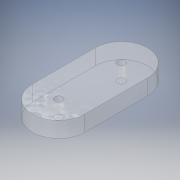
# Autodesk Inventor part: case_usb_cap
Saved by Autodesk Inventor 2019 (Build 230136000, 136)
## iProperties
Created: 2019-02-02
Part Number: case_usb_cap
Material: Acrylic, Clear
Document SubType Name: Modeling
Designer: suchanek
Density: 1.19 g/cm^3
Appearance: Transparent - Clear
Author: suchanek
Autodesk Inventor part; units mm, degrees
ref_plane "YZ Plane" through (0, 0, 0) normal (1, 0, 0) x (0, 1, 0)
ref_plane "XZ Plane" through (0, 0, 0) normal (0, 1, 0) x (-1, 0, 0)
ref_plane "XY Plane" through (0, 0, 0) normal (0, 0, 1) x (1, 0, 0)
sketch "Sketch1" plane through (0, 0, 0) normal (0, 1, 0) x (-1, 0, 0)
  line L0 (0, 0) -> (-5.6352, 0)
  line L1 (-5.6352, 0) -> (0, 0)
  line L2 (0, 0) -> (0, 8.7024)
  line L3 (6.5, 14) -> (-6.5, 14)
  line L4 (-6.5, 14) -> (-6.5, 0)
  line L5 (-6.5, 0) -> (6.5, 0)
  line L6 (6.5, 0) -> (6.5, 14)
  circle A0 centre (0, -5) radius 1.5
  circle A1 centre (0, 19) radius 1.5
  line L7 (0, 19) -> (0, -5)
  line L8 (0, 19) -> (0, -5) construction
  line L9 (-10, 19) -> (-10, -5)
  line L10 (10, -5) -> (10, 19)
  arc A2 (10, 19) -> (-10, 19) centre (0, 19) ccw
  arc A3 (-10, -5) -> (10, -5) centre (0, -5) ccw
  point P0 (0, -8.7024)
  point P1 (0, 7)
  dimension "d25" = 13
  dimension "d26" = 14
  dimension "d30" = 5
  dimension "d31" = 5
  dimension "d32" = 3
  dimension "d33" = 20
  constraints: 24 end point, 5 equal length, 4 centre point, 4 point on circle, 4 tangent, 2 horizontal, 2 midpoint, 2 vertical, 1 equal radius, 1 perpendicular, 1 point on line, 1 symmetric about line, 1 other
  measures "d25" distance of L3.start L3.end
  measures "d26" distance of L5.end L3.start
  measures "d30" distance from line of L5 L7.end
  measures "d31" distance from line of L3 L7.start
  measures "d32" diameter of A0
  measures "d33" diameter of A3
extrude "Extrusion1" add sketch "Sketch1" along normal blind 6 contours L0 L5 L4 L3 L7 L2 | L2 L7 L3 L6 L5 | A2 L10 A3 L9
body "Solid1"
